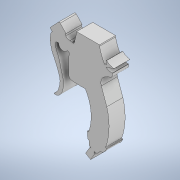
# Autodesk Inventor part: Handel
Saved by Autodesk Inventor 2021 (Build 250183000, 183)
## iProperties
Created: 2021-03-31
Part Number: Handel
Material: Generic
Document SubType Name: Modeling
Designer: newic
Density: 1 g/cm^3
Appearance: Default
Author: newic
Autodesk Inventor part; units mm, degrees
ref_plane "YZ Plane" through (0, 0, 0) normal (1, 0, 0) x (0, 1, 0)
ref_plane "XZ Plane" through (0, 0, 0) normal (0, 1, 0) x (-1, 0, 0)
ref_plane "XY Plane" through (0, 0, 0) normal (0, 0, 1) x (1, 0, 0)
sketch "Sketch1" plane through (0, 0, 0) normal (0, 1, 0) x (-1, 0, 0)
  line L0 (0, 0) -> (203.2, 0)
  line L1 (203.2, 0) -> (203.2, -50.8)
  line L2 (203.2, -50.8) -> (0, -50.8)
  line L3 (0, -50.8) -> (0, 0)
  dimension "d0" = 203.2
  dimension "d1" = 50.8
  constraints: 8 end point, 2 parallel, 1 horizontal, 1 perpendicular
  measures "d0" distance of L1.end L2.end
  measures "d1" distance of L0.end L1.end
extrude "Extrusion1" add sketch "Sketch1" along normal blind 508
sketch "Sketch2" plane through (-203.2, 0, 0) normal (0, 0, 1) x (1, 0, 0)
  line L0 (-1009.7972, -154.4296) -> (-1009.7972, 1866.7607) construction
  line L1 (-1009.7972, 1866.7607) -> (419.0943, 1866.7607) construction
  line L2 (419.0943, 1866.7607) -> (419.0943, -154.4296) construction
  line L3 (419.0943, -154.4296) -> (-1009.7972, -154.4296) construction
  line L4 (0, 0) -> (203.2, 0) projected
  line L5 (203.2, 0) -> (203.2, 508) projected
  line L6 (0, 508) -> (203.2, 508) projected
  line L7 (0, 0) -> (0, 508) projected
  line L8 (91.0468, 361.3752) -> (91.0468, 310.5752)
  line L9 (82.8238, 445.0668) -> (164.8756, 445.0668)
  line L10 (82.8238, 445.0668) -> (82.8238, 441.2568)
  line L11 (82.8238, 441.2568) -> (78.3034, 410.5475)
  line L12 (3.1885, 415.742) -> (28.6178, 442.8078)
  arc A0 (33.8054, 442.3137) -> (28.6178, 442.8078) centre (30.845, 438.7121) ccw
  line L13 (33.8054, 442.3137) -> (52.0865, 422.679)
  arc A1 (50.947, 421.5065) -> (52.0865, 422.679) centre (51.4874, 422.1212) ccw
  arc A2 (50.947, 421.5065) -> (51.4874, 416.0051) centre (55.5553, 419.182) ccw
  arc A3 (51.4874, 416.0051) -> (64.6602, 409.968) centre (64.1216, 426.1827) ccw
  arc A4 (64.6602, 409.968) -> (72.3842, 409.6129) centre (75.5655, 562.982) ccw
  line L14 (72.3842, 409.6129) -> (72.7931, 408.7008)
  line L15 (73.3725, 408.3255) -> (75.8775, 408.3255)
  line L16 (76.5125, 408.9605) -> (76.5125, 409.9125)
  line L17 (77.1475, 410.5475) -> (78.3034, 410.5475)
  arc A5 (3.1885, 415.742) -> (5.4367, 409.6129) centre (9.434, 414.556) ccw
  line L18 (5.4367, 409.6129) -> (8.691, 406.5553)
  spline S0 degree 4 poles (15.5201, 239.8196) (16.8088, 239.4457) (22.2143, 238.5217) (25.0184, 240.0183) (32.0544, 244.3487) (34.4528, 247.2114) (38.2362, 253.0254) (39.4949, 254.6178) (40.8081, 260.7252) (42.2911, 264.573) (43.2228, 269.9771) (44.2315, 274.0691) (43.7086, 278.7778) (43.7093, 287.4457) (44.2577, 292.9337) (39.7923, 300.7001) (40.6138, 305.0304) (37.8045, 312.1576) (36.387, 317.3125) (35.2527, 325.456) (32.7974, 331.6613) (31.5402, 338.9882) (29.5346, 344.404) (27.997, 348.4567) (25.6979, 355.6999) (23.1094, 359.4876) (22.0489, 364.3007) (19.5426, 368.9014) (19.5773, 373.6048) (19.0978, 377.4879) (18.7743, 382.1397) (20.2401, 383.7389) (24.9116, 387.1073) (25.8563, 385.5015) (28.6178, 385.4406) knots 0.003031 0.003031 0.003031 0.003031 0.003031 0.065124 0.094335 0.124297 0.15306 0.181334 0.209678 0.237549 0.266399 0.294874 0.325518 0.357367 0.391669 0.426118 0.459425 0.492234 0.525217 0.55995 0.595217 0.629963 0.662677 0.695168 0.726092 0.756547 0.787271 0.816351 0.845129 0.873096 0.898006 0.921739 0.943653 1 1 1 1 1
  arc A6 (28.6178, 385.3922) -> (55.2274, 377.6762) centre (42.9474, 385.0684) ccw
  arc A7 (62.6643, 372.4517) -> (55.2274, 377.6762) centre (57.4338, 372.9116) ccw
  arc A8 (60.9828, 365.9357) -> (62.6643, 372.4517) centre (52.8641, 371.5058) ccw
  line L19 (60.9828, 365.9357) -> (60.9828, 315.3134)
  arc A9 (60.9828, 315.3134) -> (70.3393, 303.6713) centre (71.0171, 313.7969) ccw
  arc A10 (70.3393, 303.6713) -> (113.1631, 302.3324) centre (101.1601, 603.9241) ccw
  arc A11 (123.8497, 190.1927) -> (113.1631, 302.3324) centre (1.241, 235.0874) ccw
  line L20 (123.8497, 190.1927) -> (120.8096, 190.1927)
  arc A12 (119.5397, 188.9096) -> (121.692, 168.7658) centre (225.1316, 190.0046) ccw
  arc A13 (121.692, 168.7658) -> (125.7984, 166.1505) centre (127.0056, 172.5776) ccw
  arc A14 (125.7984, 166.1505) -> (125.7238, 153.1608) centre (181.0937, 159.3377) ccw
  arc A15 (126.3685, 152.1917) -> (130.2735, 150.6655) centre (133.9364, 165.7954) ccw
  line L21 (130.5187, 150.1133) -> (129.4814, 148.2036)
  line L22 (141.1844, 141.9868) -> (142.5007, 144.4102)
  line L23 (128.9324, 148.0704) -> (127.6667, 148.9308)
  line L24 (127.6667, 148.9308) -> (114.0109, 126.1672)
  line L25 (114.0109, 126.1672) -> (130.0198, 116.5635)
  line L26 (130.0198, 116.5635) -> (143.7417, 140.1643)
  line L27 (143.7417, 140.1643) -> (141.3374, 141.4701)
  arc A16 (142.9491, 144.592) -> (148.5832, 143.2595) centre (155.2179, 183.8889) ccw
  arc A17 (149.6071, 143.5424) -> (161.2323, 155.4653) centre (94.1497, 209.2439) ccw
  arc A18 (161.2323, 155.4653) -> (166.5802, 154.3151) centre (168.0019, 173.9337) ccw
  arc A19 (166.5802, 154.3151) -> (180.6122, 171.592) centre (146.7932, 184.7226) ccw
  line L28 (179.7686, 173.2752) -> (177.4008, 173.9337)
  arc A20 (177.4008, 173.9337) -> (181.0937, 286.8185) centre (5.6168, 236.0561) ccw
  arc A21 (181.0937, 286.8185) -> (163.8812, 335.3453) centre (-102888.6862, -36244.7818) ccw
  arc A22 (179.2557, 367.7738) -> (163.8812, 335.3453) centre (187.8343, 343.8479) ccw
  arc A23 (193.4158, 373.3706) -> (179.2557, 367.7738) centre (200.4596, 334.8383) ccw
  arc A24 (193.4158, 373.3706) -> (199.2756, 387.3462) centre (185.7129, 384.8166) ccw
  arc A25 (178.9608, 394.2318) -> (198.6377, 387.8647) centre (197.962, 419.3645) ccw
  arc A26 (178.9608, 394.2318) -> (188.9808, 398.6669) centre (178.0127, 409.9102) ccw
  arc A27 (174.1015, 400.2668) -> (181.7268, 402.2309) centre (174.336, 415.1406) ccw
  arc A28 (179.2557, 412.3668) -> (178.9608, 403.6352) centre (199.9989, 407.2955) ccw
  arc A29 (180.6557, 413.0757) -> (179.2557, 412.3668) centre (180.4786, 411.6887) ccw
  line L29 (203.2, 0) -> (203.2, 508) projected
  arc A30 (180.6557, 413.0757) -> (202.9842, 401.9518) centre (215.2587, 454.5607) ccw
  arc A31 (189.8262, 399.9702) -> (202.9886, 401.7295) centre (194.9417, 411.8158) ccw
  arc A32 (178.9608, 403.6352) -> (181.7268, 402.2309) centre (184.0382, 410.2093) ccw
  arc A33 (188.9808, 398.6669) -> (189.8262, 399.9702) centre (183.7448, 402.989) ccw
  arc A34 (165.0276, 445.0668) -> (174.1015, 400.2668) centre (242.9441, 437.5293) ccw
  line L30 (90.7622, 445.0668) -> (152.9922, 445.0668)
  line L31 (90.7622, 445.0668) -> (85.6822, 445.0668)
  line L32 (152.9922, 445.0668) -> (158.0722, 445.0668)
  line L33 (85.6822, 445.0668) -> (85.6822, 441.2568)
  line L34 (158.0722, 445.0668) -> (158.0722, 441.2568)
  line L35 (78.3034, 410.5475) -> (85.6822, 441.2568)
  arc A35 (158.0722, 441.2568) -> (174.1015, 400.2668) centre (288.0565, 468.4585) ccw
  arc A36 (8.691, 406.5553) -> (3.4657, 396.6298) centre (18.3173, 395.1494) ccw
  arc A37 (3.4657, 396.6298) -> (2.4343, 378.256) centre (68.407, 383.7683) ccw
  arc A38 (2.4343, 378.256) -> (5.4367, 362.1067) centre (52.357, 379.1838) ccw
  arc A39 (5.4367, 362.1067) -> (13.5124, 340.6245) centre (71.1081, 374.5351) ccw
  arc A40 (30.6004, 298.6134) -> (13.5124, 340.6245) centre (-278.621, 197.3185) ccw
  arc A41 (29.5123, 262.9087) -> (30.6004, 298.6134) centre (-19.3049, 282.2654) ccw
  arc A42 (22.6286, 249.4143) -> (29.5123, 262.9087) centre (6.8723, 265.9547) ccw
  arc A43 (14.0107, 240.388) -> (19.4545, 245.6115) centre (7.0812, 253.058) ccw
  line L36 (14.0107, 240.388) -> (15.5201, 239.8196)
  arc A44 (19.4545, 245.6115) -> (22.6286, 249.4143) centre (7.9177, 258.4673) ccw
  arc A45 (120.8096, 190.1927) -> (119.5397, 188.9096) centre (120.8096, 188.9227) ccw
  arc A46 (180.6122, 171.592) -> (179.7686, 173.2752) centre (179.4283, 172.0516) ccw
  arc A47 (125.7238, 153.1608) -> (126.3685, 152.1917) centre (126.9859, 153.3016) ccw
  arc A48 (148.5832, 143.2595) -> (149.6071, 143.5424) centre (148.7879, 144.5129) ccw
  arc A49 (77.1475, 410.5475) -> (76.5125, 409.9125) centre (77.1475, 409.9125) ccw
  arc A50 (75.8775, 408.3255) -> (76.5125, 408.9605) centre (75.8775, 408.9605) ccw
  arc A51 (72.7931, 408.7008) -> (73.3725, 408.3255) centre (73.3725, 408.9605) ccw
  arc A52 (199.2756, 387.3462) -> (198.6377, 387.8647) centre (198.6514, 387.2298) ccw
  arc A53 (128.9324, 148.0704) -> (129.4814, 148.2036) centre (129.1466, 148.3855) ccw
  arc A54 (130.5187, 150.1133) -> (130.2735, 150.6655) centre (130.1839, 150.2952) ccw
  arc A55 (142.9491, 144.592) -> (142.5007, 144.4102) centre (142.8355, 144.2283) ccw
  arc A56 (141.1844, 141.9868) -> (141.3374, 141.4701) centre (141.5193, 141.805) ccw
  line L37 (0, 508) -> (203.2, 508) projected
  line L38 (0, 0) -> (203.2, 0)
  line L39 (203.2, 0) -> (203.2, 508)
  line L40 (203.2, 508) -> (0, 508)
  line L41 (0, 508) -> (0, 0)
  line L42 (-38.4114, -22.1762) -> (215.2587, -22.1762)
  line L43 (215.2587, -22.1762) -> (215.2587, 525.9486)
  line L44 (215.2587, 525.9486) -> (-38.4114, 525.9486)
  line L45 (-38.4114, 525.9486) -> (-38.4114, -22.1762)
  arc A57 (202.9886, 401.7295) -> (202.9842, 401.9518) centre (202.434, 401.8295) ccw
  arc A58 (129.7947, 116.5977) -> (130.1754, 116.6319) centre (129.9273, 117.2579) ccw
  arc A59 (114.0109, 126.2343) -> (114.0764, 126.0499) centre (114.2818, 126.2267) ccw
  arc A60 (127.8034, 148.9025) -> (127.5664, 148.8739) centre (127.7294, 148.5201) ccw
  arc A61 (143.7417, 140.0619) -> (143.7168, 140.2485) centre (143.0075, 140.0588) ccw
  arc A62 (161.1649, 155.4653) -> (161.2979, 155.4653) centre (161.2314, 156.6615) ccw
  arc A63 (125.8139, 166.1055) -> (125.7642, 166.1871) centre (125.6185, 166.0422) ccw
  arc A64 (177.4008, 174.1226) -> (177.4291, 173.8722) centre (177.8671, 174.0484) ccw
  line L46 (4.4484, 243.0319) -> (26.5918, 236.6072) construction
  arc A65 (11.614, 243.7681) -> (20.933, 241.0643) centre (17.1097, 245.2984) ccw construction
  arc A66 (28.6228, 385.3615) -> (28.6024, 385.4463) centre (28.1517, 385.2928) ccw
  point P0 (22.733, 239.4297)
  point P1 (26.6602, 241.0832)
  point P2 (31.5226, 244.3292)
  point P3 (34.7953, 247.9041)
  point P4 (38.0237, 252.6342)
  point P5 (39.3832, 255.1885)
  point P6 (40.8017, 260.1413)
  point P7 (42.1826, 264.8849)
  point P8 (43.2557, 269.8303)
  point P9 (43.8951, 273.7708)
  point P10 (43.8576, 278.4185)
  point P11 (43.8057, 286.7131)
  point P12 (43.2015, 293.5213)
  point P13 (40.6807, 300.6004)
  point P14 (39.9373, 305.3846)
  point P15 (38.1513, 311.5527)
  point P16 (36.5478, 317.4053)
  point P17 (34.987, 325.0557)
  point P18 (32.9436, 332.2254)
  point P19 (31.2101, 339.282)
  point P20 (29.5512, 344.3326)
  point P21 (27.9441, 348.7991)
  point P22 (25.4503, 355.4375)
  point P23 (23.3311, 359.8915)
  point P24 (21.7513, 364.2973)
  point P25 (20.0116, 369.1013)
  point P26 (19.4596, 373.7548)
  point P27 (19.0784, 378.2733)
  point P28 (19.1595, 381.9509)
  point P29 (20.142, 383.4352)
  point P30 (22.8222, 385.3072)
  point P31 (25.2415, 385.9029)
  point P32 (119.5342, 190.1927)
  point P33 (130.7591, 150.5561)
  point P34 (142.6507, 144.6864)
  point P35 (181.0937, 172.9067)
  point P36 (177.4059, 173.9476)
  point P37 (177.4097, 173.9312)
  point P38 (161.2373, 155.4635)
  point P39 (161.2308, 155.4635)
  point P40 (125.7975, 166.143)
  point P41 (125.7923, 166.1517)
  point P42 (28.6178, 385.39)
  point P43 (28.6042, 385.4409)
  dimension "d21" = 50.8
  dimension "d50" = 3.81
  dimension "d55" = 82.0518
  dimension "d56" = 62.23
  dimension "d57" = 5.08
  dimension "d58" = 5.08
  dimension "d63" = 1.27
  dimension "d64" = 1.27
  dimension "d65" = 0.635
  dimension "d66" = 0.381
  constraints: 140 point on circle, 74 end point, 67 centre point, 27 tangent, 8 equal radius, 8 point on line, 6 vertical, 5 horizontal, 4 parallel, 4 perpendicular, 2 midpoint, 40 other
  measures "d21" distance of L8.start L8.end
  measures "d50" distance of L9.start L10.end
  measures "d55" distance of L9.start L9.end
  measures "d56" distance of L30.start L30.end
  measures "d57" distance of L30.start L31.end
  measures "d58" distance of L30.end L32.end
  measures "d63" radius of A45
  measures "d64" radius of A47
  measures "d65" radius of A49
  measures "d66" radius of A53
extrude "Extrusion2" cut sketch "Sketch2" against normal blind 508 contours L7 L6 L5 L4 | L9 L33 L35 L11 L10 | L45 L44 L43 L42
body "Solid1"
